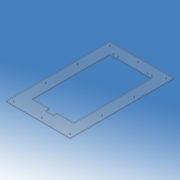
# Autodesk Inventor part: NASA-20-EBOX-T
Saved by Autodesk Inventor 2020 (Build 240168000, 168)
## iProperties
Created: 2019-09-23
Part Number: NASA-20-EBOX-T
Material: Polycarbonate, Clear
Document SubType Name: Modeling
Designer: mpark
Density: 1.2 g/cm^3
Appearance: Polycarbonate - Clear
Author: mpark
Autodesk Inventor part; units mm, degrees
ref_plane "YZ Plane" through (0, 0, 0) normal (1, 0, 0) x (0, 1, 0)
ref_plane "XZ Plane" through (0, 0, 0) normal (0, 1, 0) x (-1, 0, 0)
ref_plane "XY Plane" through (0, 0, 0) normal (0, 0, 1) x (1, 0, 0)
sketch "Sketch1" plane through (0, 0, 0) normal (0, 1, 0) x (-1, 0, 0)
  line L0 (107.95, -174.625) -> (-107.95, -174.625)
  line L1 (-107.95, -174.625) -> (-107.95, 174.625)
  line L2 (-107.95, 174.625) -> (107.95, 174.625)
  line L3 (107.95, 174.625) -> (107.95, -174.625)
  line L4 (107.95, -174.625) -> (-107.95, 174.625) construction
  line L5 (-107.95, -174.625) -> (107.95, 174.625) construction
  point P0 (0, 0)
  dimension "d0" = 215.9
  dimension "d1" = 349.25
  constraints: 12 end point, 2 midpoint, 2 parallel, 1 horizontal, 1 perpendicular
  measures "d0" distance of L1.end L2.end
  measures "d1" distance of L0.end L1.end
extrude "Thickness" add sketch "Sketch1" along normal blind 3.175
sketch "Cutout Sketch" plane through (0, 3.175, 0) normal (0, 1, 0) x (1, 0, 0)
  line L0 (107.95, -174.625) -> (107.95, 174.625) projected
  line L1 (107.95, 174.625) -> (-107.95, 174.625) projected
  line L2 (-107.95, 174.625) -> (-107.95, -174.625) projected
  line L3 (-107.95, -174.625) -> (107.95, -174.625) projected
  line L4 (-69.85, 136.525) -> (69.85, 136.525)
  line L5 (69.85, 136.525) -> (69.85, -123.825)
  line L6 (69.85, -123.825) -> (-69.85, -123.825)
  line L7 (-69.85, -123.825) -> (-69.85, 136.525)
  point P0 (0, 0)
  dimension "d4" = 38.1
  dimension "d8" = 38.1
  dimension "d9" = 50.8
  dimension "d10" = 38.1
  constraints: 8 end point, 2 parallel, 1 horizontal, 1 perpendicular
  measures "d4" distance between parallel lines of L7 L2
  measures "d8" distance between parallel lines of L5 L0
  measures "d9" distance between parallel lines of L3 L6
  measures "d10" distance between parallel lines of L1 L4
extrude "Cutout" cut sketch "Cutout Sketch" against normal blind 25.4 contours L4 L5 L6 L7
sketch "Sketch3" plane through (0, 3.175, 0) normal (0, 1, 0) x (1, 0, 0)
  line L0 (69.85, 136.525) -> (69.85, -123.825) projected
  line L1 (69.85, -123.825) -> (-69.85, -123.825) projected
  line L2 (-69.85, -123.825) -> (-69.85, 136.525) projected
  line L3 (-69.85, 136.525) -> (69.85, 136.525) projected
  line L4 (107.95, 174.625) -> (-107.95, 174.625) projected
  line L5 (-107.95, 174.625) -> (-107.95, -174.625) projected
  line L6 (-107.95, -174.625) -> (107.95, -174.625) projected
  line L7 (107.95, -174.625) -> (107.95, 174.625) projected
  line L8 (12.7, -136.525) -> (-12.7, -136.525)
  line L9 (-12.7, -136.525) -> (-12.7, -123.825)
  line L10 (-12.7, -123.825) -> (12.7, -123.825)
  line L11 (12.7, -123.825) -> (12.7, -136.525)
  point P0 (0, 0)
  point P1 (0, -136.525)
  point P2 (0, -123.825)
  dimension "d11" = 25.4
  dimension "d12" = 12.7
  constraints: 8 end point, 2 midpoint, 2 parallel, 1 horizontal, 1 perpendicular, 1 point on line, 1 vertical alignment
  measures "d11" distance of L8.start L8.end
  measures "d12" distance between parallel lines of L1 L8
extrude "Extrusion3" cut sketch "Sketch3" against normal blind 25.4 contours L11 L8 L9 L1
sketch "Sketch4" plane through (0, 3.175, 0) normal (0, 1, 0) x (1, 0, 0)
  circle A0 centre (-65.0875, 144.0656) radius 1.75 projected
  circle A1 centre (65.0875, 144.0656) radius 1.75 projected
  circle A2 centre (49.2125, 144.0656) radius 1.75 projected
  circle A3 centre (-49.2125, 144.0656) radius 1.75 projected
  line L0 (-82.55, 136.525) -> (82.55, 136.525) projected
  line L1 (82.55, 136.525) -> (82.55, -136.525) projected
  line L2 (82.55, -136.525) -> (-82.55, -136.525) projected
  line L3 (-82.55, -136.525) -> (-82.55, 136.525) projected
  line L4 (107.95, 174.625) -> (-107.95, 174.625) projected
  line L5 (-107.95, 174.625) -> (-107.95, -174.625) projected
  line L6 (-107.95, -174.625) -> (107.95, -174.625) projected
  line L7 (107.95, -174.625) -> (107.95, 174.625) projected
  circle A4 centre (-95.25, -53.975) radius 1.75 projected
  circle A5 centre (0, -161.925) radius 1.75 projected
  circle A6 centre (95.25, -53.975) radius 1.75 projected
  circle A7 centre (95.25, -161.925) radius 1.75 projected
  circle A8 centre (-95.25, -161.925) radius 1.75 projected
  circle A9 centre (-95.25, 161.925) radius 1.75 projected
  circle A10 centre (95.25, 161.925) radius 1.75 projected
  circle A11 centre (95.25, 53.975) radius 1.75 projected
  circle A12 centre (0, 161.925) radius 1.75 projected
  circle A13 centre (-95.25, 53.975) radius 1.75 projected
  point P0 (0, 0)
hole "Hole1" at (65.0875, 3.175, -144.0656) at (49.2125, 3.175, -144.0656) at (-49.2125, 3.175, -144.0656) at (-65.0875, 3.175, -144.0656) direction (0, -1, 0) diameter 3.5 end through all
sketch "Sketch5" plane through (0, 3.175, 0) normal (0, 1, 0) x (1, 0, 0)
  circle A0 centre (-95.25, -53.975) radius 1.75 projected
  circle A1 centre (0, -161.925) radius 1.75 projected
  circle A2 centre (95.25, -53.975) radius 1.75 projected
  circle A3 centre (95.25, -161.925) radius 1.75 projected
  circle A4 centre (-95.25, -161.925) radius 1.75 projected
  circle A5 centre (-95.25, 161.925) radius 1.75 projected
  circle A6 centre (95.25, 161.925) radius 1.75 projected
  circle A7 centre (95.25, 53.975) radius 1.75 projected
  circle A8 centre (0, 161.925) radius 1.75 projected
  circle A9 centre (-95.25, 53.975) radius 1.75 projected
  circle A10 centre (-65.0875, 144.0656) radius 1.75 projected
  circle A11 centre (65.0875, 144.0656) radius 1.75 projected
  circle A12 centre (49.2125, 144.0656) radius 1.75 projected
  circle A13 centre (-49.2125, 144.0656) radius 1.75 projected
  line L0 (-82.55, 136.525) -> (82.55, 136.525) projected
  line L1 (82.55, 136.525) -> (82.55, -136.525) projected
  line L2 (82.55, -136.525) -> (-82.55, -136.525) projected
  line L3 (-82.55, -136.525) -> (-82.55, 136.525) projected
  line L4 (107.95, 174.625) -> (-107.95, 174.625) projected
  line L5 (-107.95, 174.625) -> (-107.95, -174.625) projected
  line L6 (-107.95, -174.625) -> (107.95, -174.625) projected
  line L7 (107.95, -174.625) -> (107.95, 174.625) projected
  point P0 (0, 0)
hole "Hole2" at (-95.25, 3.175, 161.925) at (0, 3.175, 161.925) at (95.25, 3.175, 161.925) at (95.25, 3.175, 53.975) at (95.25, 3.175, -53.975) at (95.25, 3.175, -161.925) at (0, 3.175, -161.925) at (-95.25, 3.175, -161.925) at (-95.25, 3.175, -53.975) at (-95.25, 3.175, 53.975) direction (0, -1, 0) diameter 3.5 end through all
body "Solid1"
